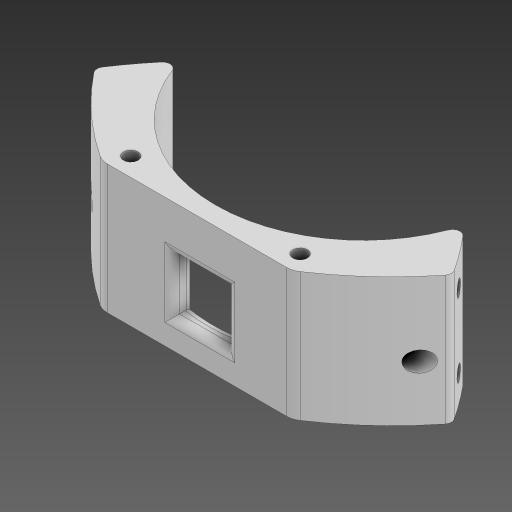
# Autodesk Inventor part: ball_solenoid
Saved by Autodesk Inventor 2023 (Build 270158000, 158)
## iProperties
Created: 2025-06-23
Part Number: ball_solenoid
Material: Типовые
Document SubType Name: Modeling
Designer: daa
Density: 1 g/cm^3
Appearance: По умолчанию
Author: daa
Autodesk Inventor part; units mm, degrees
ref_plane "YZ Plane" through (0, 0, 0) normal (1, 0, 0) x (0, 1, 0)
ref_plane "XZ Plane" through (0, 0, 0) normal (0, 1, 0) x (-1, 0, 0)
ref_plane "XY Plane" through (0, 0, 0) normal (0, 0, 1) x (1, 0, 0)
sketch "Эскиз1" plane through (0, 0, 0) normal (0, 1, 0) x (-1, 0, 0)
  line L0 (-24.3583, 67.9739) -> (24.3787, 67.9739)
  arc A0 (38.6021, 33.9735) -> (-38.5819, 33.9735) centre (0.0101, 22.7957) ccw
  arc A1 (36.6633, -21.4663) -> (-36.0003, -21.4663) centre (0.3315, -28.4663) ccw
  line L1 (36.6633, -21.4663) -> (-36.0003, -21.4663)
  circle A2 centre (23.0101, 62.9739) radius 2
  arc A3 (38.6021, 33.9735) -> (48.6021, 47.1269) centre (-38.9267, 103.2938) ccw
  circle A4 centre (-22.9899, 62.9739) radius 2
  arc A5 (-48.5819, 47.1263) -> (-38.5819, 33.9735) centre (38.9455, 103.2953) ccw
  arc A6 (-27.1271, 67.1373) -> (-48.5819, 47.1263) centre (22.7111, -7.8037) ccw
  arc A7 (48.6021, 47.1269) -> (27.1475, 67.1373) centre (-22.6902, -7.8041) ccw
  arc A8 (27.1475, 67.1373) -> (24.3787, 67.9739) centre (24.3787, 62.9739) ccw
  arc A9 (-24.3583, 67.9739) -> (-27.1271, 67.1373) centre (-24.3583, 62.9739) ccw
  line L2 (38.6021, 33.9735) -> (-38.5819, 33.9735)
  point P0 (0, 0)
  point P1 (0, 0)
  point P2 (-25.8456, 67.9739)
  point P3 (0.0102, 67.9739)
  point P4 (0, 0)
  point P5 (25.866, 67.9739)
  point P6 (-25.8046, 67.7601)
  point P7 (25.8249, 67.7602)
  point P8 (0.0101, 62.9739)
  point P9 (0.0101, 33.9735)
  dimension "d0" = 72.6636
  dimension "d1" = 37
  dimension "d2" = 10
  dimension "d4" = 5
  dimension "d5" = 5
  dimension "d6" = 90
  dimension "d7" = 90
  dimension "d8" = 5
  dimension "d98" = 10
  dimension "d105" = 77.184
  dimension "d108" = 4
  dimension "d109" = 4
  dimension "d111" = 40.1782
  dimension "d112" = 5
  constraints: 21 point on circle, 10 centre point, 6 end point, 4 tangent, 3 horizontal, 2 midpoint, 2 point on line, 1 equal radius
  measures "d0" distance of L1.start L1.end
  measures "d1" radius of A1
  measures "d2" horizontal distance of A6.end L2.end
  measures "d4" vertical distance of point (25.866, 67.974) A2.centre
  measures "d5" vertical distance of point (-25.846, 67.974) A4.centre
  measures "d6" radius of A6
  measures "d7" radius of A7
  measures "d8" radius of A8
  measures "d98" horizontal distance of L2.start A7.start
  measures "d105" distance of L2.end L2.start
  measures "d108" diameter of A2
  measures "d109" diameter of A4
  measures "d111" radius of A0
  measures "d112" distance of point (0.01, 67.974) point (0.01, 62.974)
extrude "Выдавливание1" add sketch "Эскиз1" along normal blind 35 contours L0 A8 A7 A3 A0 A5 A6 A9
sketch "Эскиз7" plane through (-24.3787, 0, 67.9739) normal (0, 0, 1) x (1, 0, 0)
  line L0 (17.61, 22.5) -> (32.61, 22.5)
  line L1 (32.61, 22.5) -> (32.61, 7.5)
  line L2 (32.61, 7.5) -> (17.61, 7.5)
  line L3 (17.61, 7.5) -> (17.61, 22.5)
  line L4 (0, 35) -> (48.737, 35) projected
  line L5 (0, 0) -> (0, 35) projected
  point P0 (24.3787, 0)
  dimension "d40" = 15
  dimension "d41" = 15
  dimension "d42" = 12.5
  dimension "d43" = 17.61
  constraints: 8 end point, 2 parallel, 1 horizontal, 1 perpendicular
  measures "d40" distance of L1.end L2.end
  measures "d41" distance of L0.end L1.end
  measures "d42" distance between parallel lines of L4 L0
  measures "d43" distance between parallel lines of L5 L3
extrude "Выдавливание5" cut sketch "Эскиз7" against normal blind 48
fillet "Сопряжение1" radius 2 8 edges at (0.7313, 7.5, 67.9739) (-6.7687, 15, 67.9739) (0.7313, 22.5, 67.9739) (8.2313, 15, 67.9739) (8.2313, 15, 62.1195) (0.7446, 22.5, 62.9668) (-6.7687, 15, 62.4013) (0.7446, 7.5, 62.9668)
fillet "Сопряжение2" radius 2 4 edges at (48.5819, 17.5, 47.1263) (38.5819, 17.5, 33.9735) (-38.6021, 17.5, 33.9735) (-48.6021, 17.5, 47.1269)
ref_plane "РабПлоскость4" through (40.8942, 0, 36.6497) normal (0.7676891, 0, -0.6408224) x (0, 1, 0)
sketch "Эскиз9" plane through (40.8942, 0, 36.6497) normal (0.7676891, 0, -0.6408224) x (0, 1, 0)
  circle A0 centre (27.5, 6.7446) radius 2
  circle A1 centre (7.5, 6.7446) radius 2
  line L0 (35, 0) -> (35, 11.5346) projected
  line L1 (0, 11.5346) -> (35, 11.5346) projected
  point P0 (0, -54.3415)
  dimension "d49" = 4
  dimension "d50" = 4
  dimension "d51" = 20
  dimension "d52" = 7.5
  dimension "d53" = 4.79
  dimension "d54" = 4.79
  constraints: 2 centre point
  measures "d49" diameter of A0
  measures "d50" diameter of A1
  measures "d51" distance of A1.centre A0.centre
  measures "d52" distance from line of A0.centre L0
  measures "d53" distance from line of A0.centre L1
  measures "d54" distance from line of L1 A1.centre
extrude "Выдавливание6" cut sketch "Эскиз9" against normal blind 10
ref_plane "РабПлоскость9" through (-48.6155, 0, 45.3193) normal (0.8021089, 0, 0.5971778) x (0, -1, 0)
ref_plane "РабПлоскость8" through (-47.8134, 0, 45.9165) normal (0.8021089, 0, 0.5971778) x (0, -1, 0)
sketch "Эскиз12" plane through (-48.6155, 0, 45.3193) normal (0.8021089, 0, 0.5971778) x (0, -1, 0)
  circle A0 centre (-27.5, 6.7628) radius 2
  circle A1 centre (-7.5, 6.7628) radius 2
  line L0 (0, 11.5528) -> (-35, 11.5528) projected
  line L1 (-35, 11.5528) -> (-35, 0) projected
  point P0 (0, 65.3831)
  dimension "d66" = 4
  dimension "d67" = 4
  dimension "d68" = 20
  dimension "d69" = 4.79
  dimension "d70" = 4.79
  dimension "d71" = 7.5
  constraints: 2 centre point
  measures "d66" diameter of A0
  measures "d67" diameter of A1
  measures "d68" distance of A1.centre A0.centre
  measures "d69" distance from line of A0.centre L0
  measures "d70" distance from line of A1.centre L0
  measures "d71" distance from line of L1 A0.centre
extrude "Выдавливание8" cut sketch "Эскиз12" along normal blind 10
ref_plane "РабПлоскость12" through (47.6896, 0, 48.2653) normal (-0.9961947, 0, -0.0871557) x (0, -1, 0)
sketch "Эскиз14" plane through (47.6896, 0, 48.2653) normal (-0.9961947, 0, -0.0871557) x (0, -1, 0)
  circle A0 centre (-15, 4) radius 2.75
  line L0 (0, 20.5923) -> (0, 0) projected
  line L1 (-35, 0) -> (0, 0) projected
  point P0 (0, -43.9252)
  dimension "d78" = 5.5
  dimension "d79" = 15
  dimension "d80" = 4
  constraints: 1 centre point
  measures "d78" diameter of A0
  measures "d79" distance from line of A0.centre L0
  measures "d80" distance from line of L1 A0.centre
extrude "Выдавливание9" cut sketch "Эскиз14" along normal blind 43.25
ref_plane "РабПлоскость13" through (-47.7098, 0, 48.2659) normal (-0.9052218, 0, -0.4249394) x (0, 1, 0)
sketch "Эскиз16" plane through (-47.7098, 0, 48.2659) normal (-0.9052218, 0, -0.4249394) x (0, 1, 0)
  circle A0 centre (15, -4) radius 2.25
  line L0 (0, -8.3451) -> (0, 0) projected
  line L1 (0, 0) -> (35, 0) projected
  point P0 (0, 63.9651)
  dimension "d85" = 4.5
  dimension "d86" = 15
  dimension "d87" = 4
  constraints: 1 centre point
  measures "d85" diameter of A0
  measures "d86" distance from line of L0 A0.centre
  measures "d87" distance from line of A0.centre L1
extrude "Выдавливание10" cut sketch "Эскиз16" against normal blind 15.5
sketch "Эскиз17" plane through (-47.7098, 0, 48.2659) normal (-0.9052218, 0, -0.4249394) x (0, 1, 0)
  circle A0 centre (15, -4) radius 1.25
  line L0 (0, -8.3451) -> (0, 0) projected
  line L1 (0, 0) -> (35, 0) projected
  point P0 (0, 63.9651)
  dimension "d90" = 2.5
  dimension "d91" = 15
  dimension "d92" = 4
  constraints: 1 centre point
  measures "d90" diameter of A0
  measures "d91" distance from line of L0 A0.centre
  measures "d92" distance from line of A0.centre L1
extrude "Выдавливание11" cut sketch "Эскиз17" against normal blind 31.25
